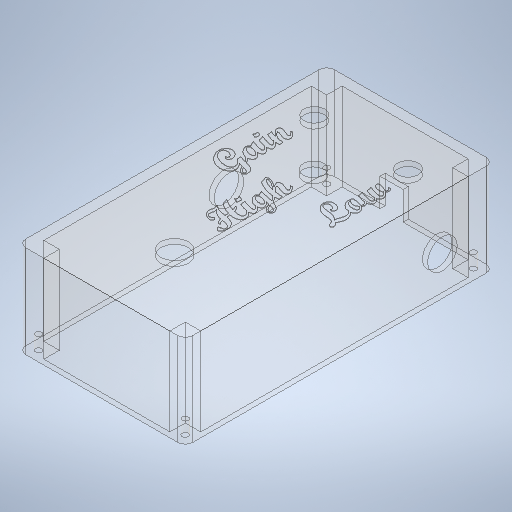
# Autodesk Inventor part: obudowa
Saved by Autodesk Inventor 2025 (Build 290162000, 162)
## iProperties
Created: 2026-04-02
Part Number: obudowa
Material: Tworzywo sztuczne PET
Document SubType Name: Modeling
Designer: zzapa
Density: 1.541 g/cm^3
Appearance: Poliwęglan — przezroczysty
Author: zzapa
Autodesk Inventor part; units mm, degrees
ref_plane "YZ Plane" through (0, 0, 0) normal (1, 0, 0) x (0, 1, 0)
ref_plane "XZ Plane" through (0, 0, 0) normal (0, 1, 0) x (-1, 0, 0)
ref_plane "XY Plane" through (0, 0, 0) normal (0, 0, 1) x (1, 0, 0)
sketch "Szkic1" plane through (0, 0, 0) normal (0, 1, 0) x (-1, 0, 0)
  line L0 (65, -120) -> (0, -120)
  line L1 (0, -120) -> (0, 0)
  line L2 (0, 0) -> (65, 0)
  line L3 (65, 0) -> (65, -120)
  dimension "d0" = 120
  dimension "d1" = 65
  constraints: 8 end point, 2 parallel, 1 coincident, 1 horizontal, 1 perpendicular
  measures "d0" distance of L2.end L0.start
  measures "d1" distance of L0.start L0.end
extrude "Gabaryt" add sketch "Szkic1" along normal blind 36
ref_plane "Konstrukcja wycięcia" through (0, 34, 0) normal (0, 1, 0) x (1, 0, 0)
sketch "Szkic2" plane through (0, 0, 0) normal (0, -1, 0) x (1, 0, 0)
  line L0 (-65, 0) -> (0, 0) projected
  line L1 (-65, -120) -> (-65, 0) projected
  line L2 (0, -120) -> (-65, -120) projected
  line L3 (0, 0) -> (0, -120) projected
  line L4 (-2, -118) -> (-63, -118)
  line L5 (-63, -118) -> (-63, -2)
  line L6 (-63, -2) -> (-2, -2)
  line L7 (-2, -2) -> (-2, -118)
  dimension "d4" = 2
  constraints: 8 end point, 3 other
  measures "d4" distance between parallel lines of L3 L7
extrude "Wydrążenie" cut sketch "Szkic2" against normal up to surface (34 mm away) contours L4 L5 L6 L7
sketch "Szkic6" plane through (0, 0, 0) normal (0, -1, 0) x (1, 0, 0)
  line L0 (-65, 0) -> (0, 0) projected
  line L1 (-8, -8) -> (0, -8)
  line L2 (0, -8) -> (0, 0)
  line L3 (0, 0) -> (-8, 0)
  line L4 (-8, 0) -> (-8, -8)
  line L5 (0, 0) -> (0, -120) projected
  line L6 (0, -120) -> (-65, -120) projected
  line L7 (-65, -120) -> (-65, 0) projected
  line L8 (0, 0) -> (0, -120) projected
  line L9 (0, -60) -> (-65, -60)
  line L10 (-32.5, 0) -> (-32.5, -120)
  line L11 (-57, -8) -> (-65, -8)
  line L12 (-65, -8) -> (-65, 0)
  line L13 (-65, 0) -> (-57, 0)
  line L14 (-57, 0) -> (-57, -8)
  line L15 (-8, -112) -> (0, -112)
  line L16 (0, -112) -> (0, -120)
  line L17 (0, -120) -> (-8, -120)
  line L18 (-8, -120) -> (-8, -112)
  line L19 (-57, -112) -> (-65, -112)
  line L20 (-65, -112) -> (-65, -120)
  line L21 (-65, -120) -> (-57, -120)
  line L22 (-57, -120) -> (-57, -112)
  point P0 (-57, -120)
  point P1 (-65, -112)
  point P2 (-57, 0)
  point P3 (-8, -120)
  point P4 (0, -112)
  point P5 (-8, 0)
  dimension "d16" = 8
  dimension "d17" = 8
  constraints: 36 end point, 9 symmetric about line, 4 midpoint, 2 parallel, 1 horizontal, 1 perpendicular
  measures "d16" distance of L1.start L1.end
  measures "d17" distance of L3.end L1.start
extrude "Materiał na insert" add sketch "Szkic6" against normal up to surface (34 mm away) contours L0 L14 L11 L7 | L0 L2 L1 L4 | L19 L22 L6 L7 | L5 L6 L18 L15
sketch "Szkic7" plane through (0, 0, 0) normal (0, -1, 0) x (1, 0, 0)
  line L0 (0, 0) -> (0, -120) projected
  line L1 (0, -60) -> (-65, -60)
  line L2 (-65, -120) -> (-65, 0) projected
  line L3 (0, -120) -> (-65, -120) projected
  line L4 (-32.5, -120) -> (-32.5, 0)
  line L5 (-65, 0) -> (0, 0) projected
  point P0 (-4, -4)
  point P1 (-61, -4)
  point P2 (-4, -116)
  point P3 (-61, -116)
  dimension "d20" = 4
  dimension "d21" = 4
  constraints: 4 end point, 4 midpoint, 3 symmetric about line
  measures "d20" horizontal distance of L0.start point (-4, -4)
  measures "d21" horizontal distance of point (-4, -4) L0.start
hole "Otwory montażowe" at (-4, 0, -4) at (-61, 0, -4) at (-4, 0, -116) at (-61, 0, -116) direction (0, 1, 0) diameter 2.4 depth 5.5
fillet "Zaokrąglenie1" radius 3 4 edges at (-65, 18, 0) (0, 18, 0) (0, 18, -120) (-65, 18, -120)
sketch "Szkic8" plane through (-65, 0, -117) normal (-1, 0, 0) x (0, 0, 1)
  line L0 (-3, 36) -> (-3, 0) projected
  line L1 (0, 0) -> (114, 0) projected
  line L2 (0, 0) -> (-3, 0) projected
  line L3 (117, 0) -> (117, 36) projected
  point P0 (37, 15)
  dimension "d30" = 15
  dimension "d39" = 80
  measures "d30" distance from line of L1 point (37, 15)
  measures "d39" distance from line of L3 point (37, 15)
hole "JACK 1" at (-65, 15, -80) direction (1, 0, 0) diameter 11.5 depth 2
sketch "Szkic9" plane through (0, 0, -3) normal (1, 0, 0) x (0, 0, -1)
  line L0 (0, 0) -> (114, 0) projected
  line L1 (-3, 36) -> (-3, 0) projected
  point P0 (97, 15)
  dimension "d40" = 15
  dimension "d41" = 100
  measures "d40" distance from line of L0 point (97, 15)
  measures "d41" distance from line of point (97, 15) L1
hole "JACK 2" at (0, 15, -100) direction (-1, 0, 0) diameter 11.5 end up to face face through (-2, 11.3333, -77.3333) facing (-1, 0, 0)
sketch "Szkic11" plane through (0, 36, 0) normal (0, 1, 0) x (1, 0, 0)
  circle A0 centre (-50.7217, 100.8782) radius 4
  circle A1 centre (-32.5, 82.3712) radius 4
  line L0 (-3, 120) -> (-62, 120) projected
  line L1 (-32.5, 120) -> (-32.5, 0)
  line L2 (-62, 0) -> (-3, 0) projected
  circle A2 centre (-14.2783, 100.8782) radius 4
  circle A3 centre (-32.5, 28.3603) radius 5.3281
  point P0 (0, 0)
  dimension "d51" = 8
  constraints: 4 centre point, 2 end point, 2 midpoint, 2 point on line, 1 equal radius, 1 symmetric about line, 1 other
  measures "d51" diameter of A0
extrude "Wyciągnięcie proste7" cut sketch "Szkic11" against normal up to surface (2 mm away)
sketch "Szkic12" plane through (-3, 0, -120) normal (0, 0, -1) x (-1, 0, 0)
  line L0 (0, 0) -> (59, 0) projected
  line L1 (30.3172, 11) -> (39.3172, 11)
  line L2 (39.3172, 11) -> (39.3172, 0)
  line L3 (39.3172, 0) -> (30.3172, 0)
  line L4 (30.3172, 0) -> (30.3172, 11)
  point P0 (-3, 0)
  point P1 (30.3172, 0)
  dimension "d54" = 11
  dimension "d55" = 9
  constraints: 8 end point, 2 parallel, 1 horizontal, 1 perpendicular, 1 point on line
  measures "d54" distance of L3.end L1.start
  measures "d55" distance of L1.start L1.end
extrude "Wyciągnięcie proste8" cut sketch "Szkic12" against normal up to surface (2 mm away)
sketch "Szkic13" plane through (0, 36, 0) normal (0, 1, 0) x (1, 0, 0)
  line L0 (-58.0791, 56.7666) -> (-58.0791, 90.8782) construction
  line L1 (-58.0791, 90.8782) -> (-43.3643, 90.8782) construction
  line L2 (-43.3643, 90.8782) -> (-43.3643, 56.7666) construction
  line L3 (-43.3643, 56.7666) -> (-58.0791, 56.7666) construction
  line L4 (-41.629, 38.2595) -> (-41.629, 72.3712) construction
  line L5 (-41.629, 72.3712) -> (-23.371, 72.3712) construction
  line L6 (-23.371, 72.3712) -> (-23.371, 38.2595) construction
  line L7 (-23.371, 38.2595) -> (-41.629, 38.2595) construction
  line L8 (-22.0376, 56.7666) -> (-22.0376, 90.8782) construction
  line L9 (-22.0376, 90.8782) -> (-6.519, 90.8782) construction
  line L10 (-6.519, 90.8782) -> (-6.519, 56.7666) construction
  line L11 (-6.519, 56.7666) -> (-22.0376, 56.7666) construction
  circle A0 centre (-50.7217, 100.8782) radius 4 projected
  circle A1 centre (-32.5, 82.3712) radius 4 projected
  circle A2 centre (-14.2783, 100.8782) radius 4 projected
  line L12 (-50.7217, 100.8782) -> (-50.7217, 90.8782)
  line L13 (-32.5, 82.3712) -> (-32.5, 72.3712)
  line L14 (-14.2783, 100.8782) -> (-14.2783, 90.8782)
  spline S0 degree 2 poles (-49.1006, 73.4653) (-48.5617, 73.001) (-47.8817, 71.6743) knots 0 0 0 1 1 1
  spline S1 degree 2 poles (-47.8817, 71.6743) (-46.0492, 71.4006) (-44.0426, 69.5101) (-44.0426, 68.3326) knots 0 0 0 1 2 2 2
  spline S2 degree 2 poles (-44.0426, 68.3326) (-44.0426, 67.7688) (-44.565, 67.1303) (-45.0293, 67.1303) knots 0 0 0 1 2 2 2
  spline S3 degree 2 poles (-45.0293, 67.1303) (-46.3146, 67.1303) (-47.5169, 69.6262) knots 0 0 0 1 1 1
  spline S4 degree 2 poles (-47.5169, 69.6262) (-48.4456, 69.8832) (-49.1836, 70.132) knots 0 0 0 1 1 1
  spline S5 degree 2 poles (-49.1836, 70.132) (-48.5617, 69.6925) (-47.5998, 68.0424) (-47.5998, 67.3293) knots 0 0 0 1 2 2 2
  spline S6 degree 2 poles (-47.5998, 67.3293) (-47.5998, 66.1685) (-49.6064, 64.6345) (-51.1404, 64.6345) knots 0 0 0 1 2 2 2
  spline S7 degree 2 poles (-51.1404, 64.6345) (-52.7574, 64.6345) (-55.6595, 66.3675) (-57.4008, 69.195) (-57.4008, 70.5134) knots 0 0 0 1 2 3 3 3
  spline S8 degree 2 poles (-57.4008, 70.5134) (-57.4008, 71.6991) (-56.0492, 73.1834) (-54.9713, 73.1834) knots 0 0 0 1 2 2 2
  spline S9 degree 2 poles (-54.9713, 73.1834) (-53.8187, 73.1834) (-52.0525, 71.5167) (-52.0525, 70.4388) knots 0 0 0 1 2 2 2
  spline S10 degree 2 poles (-52.0525, 70.4388) (-52.0525, 69.8003) (-52.6744, 68.9711) (-53.1222, 68.9711) knots 0 0 0 1 2 2 2
  spline S11 degree 2 poles (-53.1222, 68.9711) (-53.4041, 68.9711) (-53.827, 69.2945) (-53.827, 69.5101) knots 0 0 0 1 2 2 2
  spline S12 degree 2 poles (-53.827, 69.5101) (-53.827, 69.7174) (-53.5865, 69.7174) knots 0 0 0 1 1 1
  spline S13 degree 2 poles (-53.5865, 69.7174) (-53.371, 69.7174) (-53.1388, 70.0325) (-53.1388, 70.2398) knots 0 0 0 1 2 2 2
  spline S14 degree 2 poles (-53.1388, 70.2398) (-53.1388, 70.787) (-54.6479, 71.7986) (-55.5103, 71.7986) knots 0 0 0 1 2 2 2
  spline S15 degree 2 poles (-55.5103, 71.7986) (-56.1239, 71.7986) (-56.8867, 71.0109) (-56.8867, 70.3973) knots 0 0 0 1 2 2 2
  spline S16 degree 2 poles (-56.8867, 70.3973) (-56.8867, 69.4603) (-55.2366, 67.719) (-52.5418, 66.6245) (-51.3229, 66.6245) knots 0 0 0 1 2 3 3 3
  spline S17 degree 2 poles (-51.3229, 66.6245) (-50.2117, 66.6245) (-48.8933, 67.5864) (-48.8933, 68.3824) knots 0 0 0 1 2 2 2
  spline S18 degree 2 poles (-48.8933, 68.3824) (-48.8933, 69.734) (-50.8005, 70.9695) knots 0 0 0 1 1 1
  line L15 (-50.8005, 70.9695) -> (-50.9829, 72.263)
  spline S19 degree 2 poles (-50.9829, 72.263) (-51.0161, 72.5035) (-50.8668, 72.5035) knots 0 0 0 1 1 1
  spline S20 degree 2 poles (-50.8668, 72.5035) (-50.8005, 72.5035) (-49.7557, 72.1386) (-48.5285, 71.8152) knots 0 0 0 1 2 2 2
  spline S21 degree 2 poles (-48.5285, 71.8152) (-49.1421, 72.8849) (-49.8967, 73.4653) knots 0 0 0 1 1 1
  line L16 (-49.8967, 73.4653) -> (-49.1006, 73.4653)
  spline S22 degree 2 poles (-46.8204, 69.4603) (-45.9249, 67.6693) (-45.0542, 67.6693) knots 0 0 0 1 1 1
  spline S23 degree 2 poles (-45.0542, 67.6693) (-44.5899, 67.6693) (-44.5899, 68.1088) knots 0 0 0 1 1 1
  spline S24 degree 2 poles (-44.5899, 68.1088) (-44.5899, 68.9794) (-46.8204, 69.4603) knots 0 0 0 1 1 1
  spline S25 degree 2 poles (-49.1006, 80.8119) (-48.0559, 79.7091) (-47.4257, 78.7555) (-47.4257, 78.3243) knots 0 0 0 1 2 2 2
  spline S26 degree 2 poles (-47.4257, 78.3243) (-47.4257, 77.2381) (-49.3494, 77.2962) knots 0 0 0 1 1 1
  spline S27 degree 2 poles (-49.3494, 77.2962) (-48.3627, 76.6079) (-47.4257, 75.4471) (-47.4257, 74.8252) knots 0 0 0 1 2 2 2
  spline S28 degree 2 poles (-47.4257, 74.8252) (-47.4257, 74.2199) (-48.5617, 73.3741) (-49.3909, 73.3741) knots 0 0 0 1 2 2 2
  spline S29 degree 2 poles (-49.3909, 73.3741) (-50.419, 73.3741) (-52.293, 74.5101) (-53.4539, 76.2845) (-53.4539, 76.9645) knots 0 0 0 1 2 3 3 3
  spline S30 degree 2 poles (-53.4539, 76.9645) (-53.4539, 77.8268) (-52.6579, 78.1668) knots 0 0 0 1 1 1
  line L17 (-52.6579, 78.1668) -> (-53.4373, 79.5847)
  line L18 (-53.4373, 79.5847) -> (-53.4373, 79.9744)
  line L19 (-53.4373, 79.9744) -> (-51.4224, 79.3608)
  spline S31 degree 2 poles (-51.4224, 79.3608) (-49.8967, 78.8882) (-49.3328, 78.8882) knots 0 0 0 1 1 1
  spline S32 degree 2 poles (-49.3328, 78.8882) (-48.7441, 78.8882) (-48.7441, 79.3111) knots 0 0 0 1 1 1
  spline S33 degree 2 poles (-48.7441, 79.3111) (-48.7441, 79.5764) (-49.3162, 80.2232) (-49.8967, 80.8119) knots 0 0 0 1 2 2 2
  line L20 (-49.8967, 80.8119) -> (-49.1006, 80.8119)
  spline S34 degree 2 poles (-48.7275, 75.7704) (-48.7275, 76.4587) (-51.0741, 77.6776) (-52.0691, 77.6776) knots 0 0 0 1 2 2 2
  spline S35 degree 2 poles (-52.0691, 77.6776) (-52.4588, 77.6776) (-52.89, 77.3293) (-52.89, 77.0391) knots 0 0 0 1 2 2 2
  spline S36 degree 2 poles (-52.89, 77.0391) (-52.89, 76.3509) (-50.5434, 75.1237) (-49.565, 75.1237) knots 0 0 0 1 2 2 2
  spline S37 degree 2 poles (-49.565, 75.1237) (-49.1918, 75.1237) (-48.7275, 75.4885) (-48.7275, 75.7704) knots 0 0 0 1 2 2 2
  spline S38 degree 2 poles (-49.1006, 84.195) (-47.4091, 82.5864) (-47.4091, 81.7821) knots 0 0 0 1 1 1
  spline S39 degree 2 poles (-47.4091, 81.7821) (-47.4091, 81.3426) (-48.3129, 80.7373) (-48.9928, 80.7373) knots 0 0 0 1 2 2 2
  spline S40 degree 2 poles (-48.9928, 80.7373) (-50.4605, 80.7373) (-53.0559, 81.7323) knots 0 0 0 1 1 1
  line L21 (-53.0559, 81.7323) -> (-53.4207, 83.4819)
  line L22 (-53.4207, 83.4819) -> (-53.4207, 83.5648)
  line L23 (-53.4207, 83.5648) -> (-51.2648, 82.8766)
  spline S41 degree 2 poles (-51.2648, 82.8766) (-49.9298, 82.4454) (-49.3577, 82.4454) knots 0 0 0 1 1 1
  spline S42 degree 2 poles (-49.3577, 82.4454) (-49.1338, 82.4454) (-48.8519, 82.6444) (-48.8519, 82.7937) knots 0 0 0 1 2 2 2
  spline S43 degree 2 poles (-48.8519, 82.7937) (-48.8519, 83.0673) (-49.2416, 83.6063) (-49.8967, 84.195) knots 0 0 0 1 2 2 2
  line L24 (-49.8967, 84.195) -> (-49.1006, 84.195)
  spline S44 degree 2 poles (-56.1073, 84.054) (-54.4572, 84.054) (-54.4572, 82.8351) knots 0 0 0 1 1 1
  spline S45 degree 2 poles (-54.4572, 82.8351) (-54.4572, 82.2464) (-54.8137, 81.8235) knots 0 0 0 1 1 1
  spline S46 degree 2 poles (-54.8137, 81.8235) (-55.419, 82.2215) (-56.1736, 82.4454) knots 0 0 0 1 1 1
  spline S47 degree 2 poles (-56.1736, 82.4454) (-55.8419, 82.9844) (-55.8419, 83.3161) knots 0 0 0 1 1 1
  spline S48 degree 2 poles (-55.8419, 83.3161) (-55.8419, 83.6892) (-56.1073, 84.054) knots 0 0 0 1 1 1
  spline S49 degree 2 poles (-49.1089, 90.9612) (-47.4257, 89.3691) (-47.4257, 88.2331) knots 0 0 0 1 1 1
  spline S50 degree 2 poles (-47.4257, 88.2331) (-47.4257, 87.7688) (-48.0724, 87.2049) (-48.6197, 87.2049) knots 0 0 0 1 2 2 2
  spline S51 degree 2 poles (-48.6197, 87.2049) (-49.3577, 87.2049) (-50.8668, 87.8102) knots 0 0 0 1 1 1
  spline S52 degree 2 poles (-50.8668, 87.8102) (-51.6794, 88.1336) (-51.895, 88.1336) knots 0 0 0 1 1 1
  spline S53 degree 2 poles (-51.895, 88.1336) (-52.1189, 88.1336) (-52.1189, 87.9595) knots 0 0 0 1 1 1
  spline S54 degree 2 poles (-52.1189, 87.9595) (-52.1189, 87.8683) (-52.0194, 87.7107) knots 0 0 0 1 1 1
  spline S55 degree 2 poles (-52.0194, 87.7107) (-51.9282, 87.5615) (-51.754, 87.3708) knots 0 0 0 1 1 1
  spline S56 degree 2 poles (-51.754, 87.3708) (-51.5965, 87.1967) (-51.3643, 86.9894) knots 0 0 0 1 1 1
  spline S57 degree 2 poles (-51.3643, 86.9894) (-51.1736, 86.7986) (-50.9249, 86.5913) knots 0 0 0 1 1 1
  line L25 (-50.9249, 86.5913) -> (-50.4771, 86.2016)
  spline S58 degree 2 poles (-50.4771, 86.2016) (-50.1703, 85.9529) (-49.822, 85.8865) knots 0 0 0 1 1 1
  spline S59 degree 2 poles (-49.822, 85.8865) (-49.2416, 85.787) (-48.7524, 85.7456) knots 0 0 0 1 1 1
  spline S60 degree 2 poles (-48.7524, 85.7456) (-48.3875, 85.729) (-47.7656, 85.729) knots 0 0 0 1 1 1
  line L26 (-47.7656, 85.729) -> (-47.4091, 84.2033)
  spline S61 degree 2 poles (-47.4091, 84.2033) (-48.3378, 84.1287) (-48.7938, 84.1287) knots 0 0 0 1 1 1
  spline S62 degree 2 poles (-48.7938, 84.1287) (-49.9049, 84.1287) (-51.8867, 84.6428) (-53.1305, 85.2149) knots 0 0 0 1 2 2 2
  line L27 (-53.1305, 85.2149) -> (-53.4539, 86.8981)
  spline S63 degree 2 poles (-53.4539, 86.8981) (-52.0277, 86.3675) (-51.2068, 86.2016) knots 0 0 0 1 1 1
  spline S64 degree 2 poles (-51.2068, 86.2016) (-52.4671, 87.3293) (-53.4373, 88.656) (-53.4373, 89.1784) knots 0 0 0 1 2 2 2
  spline S65 degree 2 poles (-53.4373, 89.1784) (-53.4373, 89.5267) (-52.9066, 89.991) (-52.5086, 89.991) knots 0 0 0 1 2 2 2
  spline S66 degree 2 poles (-52.5086, 89.991) (-51.8452, 89.991) (-50.3361, 89.4023) knots 0 0 0 1 1 1
  spline S67 degree 2 poles (-50.3361, 89.4023) (-49.2914, 88.9877) (-48.9846, 88.9877) knots 0 0 0 1 1 1
  spline S68 degree 2 poles (-48.9846, 88.9877) (-48.57, 88.9877) (-48.57, 89.3277) knots 0 0 0 1 1 1
  spline S69 degree 2 poles (-48.57, 89.3277) (-48.57, 89.8335) (-49.8967, 90.9612) knots 0 0 0 1 1 1
  line L28 (-49.8967, 90.9612) -> (-49.1089, 90.9612)
  spline S70 degree 2 poles (-30.8541, 55.5553) (-29.9834, 54.7178) (-29.1708, 53.3413) (-29.1708, 52.6199) knots 0 0 0 1 2 2 2
  spline S71 degree 2 poles (-29.1708, 52.6199) (-29.1708, 51.8073) (-30.6053, 50.6962) (-31.9818, 50.6962) knots 0 0 0 1 2 2 2
  spline S72 degree 2 poles (-31.9818, 50.6962) (-32.5539, 50.6962) (-33.4826, 50.8455) knots 0 0 0 1 1 1
  spline S73 degree 2 poles (-33.4826, 50.8455) (-33.3997, 49.809) (-33.3831, 49.5768) knots 0 0 0 1 1 1
  spline S74 degree 2 poles (-33.3831, 49.5768) (-31.1111, 49.1374) (-29.1708, 46.9566) (-29.1708, 45.5719) knots 0 0 0 1 2 2 2
  spline S75 degree 2 poles (-29.1708, 45.5719) (-29.1708, 44.552) (-30.1161, 43.2335) (-30.5556, 43.2335) knots 0 0 0 1 2 2 2
  spline S76 degree 2 poles (-30.5556, 43.2335) (-30.8789, 43.2335) (-31.7081, 44.2203) (-31.7081, 44.411) knots 0 0 0 1 2 2 2
  spline S77 degree 2 poles (-31.7081, 44.411) (-31.7081, 44.6763) (-31.1277, 44.6763) knots 0 0 0 1 1 1
  spline S78 degree 2 poles (-31.1277, 44.6763) (-29.7098, 44.6763) (-29.7098, 45.6299) knots 0 0 0 1 1 1
  spline S79 degree 2 poles (-29.7098, 45.6299) (-29.7098, 46.3347) (-31.2769, 47.2634) (-33.1012, 47.5453) knots 0 0 0 1 2 2 2
  spline S80 degree 2 poles (-33.1012, 47.5453) (-32.9851, 46.7161) (-32.2968, 45.9035) knots 0 0 0 1 1 1
  spline S81 degree 2 poles (-32.2968, 45.9035) (-32.3715, 45.8455) (-32.8856, 45.804) knots 0 0 0 1 1 1
  spline S82 degree 2 poles (-32.8856, 45.804) (-33.6899, 46.5254) (-34.005, 47.7194) knots 0 0 0 1 1 1
  spline S83 degree 2 poles (-34.005, 47.7194) (-35.1161, 47.9599) (-36.5257, 48.6896) (-37.9934, 50.1821) knots 0 0 0 1 2 2 2
  spline S84 degree 2 poles (-37.9934, 50.1821) (-37.7114, 49.4607) (-37.7114, 49.0047) knots 0 0 0 1 1 1
  spline S85 degree 2 poles (-37.7114, 49.0047) (-37.7114, 48.7145) (-38.0265, 47.8272) (-38.0265, 47.5536) knots 0 0 0 1 2 2 2
  spline S86 degree 2 poles (-38.0265, 47.5536) (-38.0265, 46.9732) (-37.1808, 46.2269) (-36.7413, 46.2269) knots 0 0 0 1 2 2 2
  spline S87 degree 2 poles (-36.7413, 46.2269) (-36.3018, 46.2269) (-35.937, 46.6913) knots 0 0 0 1 1 1
  spline S88 degree 2 poles (-35.937, 46.6913) (-35.8043, 46.9068) (-35.6882, 46.9068) knots 0 0 0 1 1 1
  spline S89 degree 2 poles (-35.6882, 46.9068) (-35.4809, 46.9068) (-34.8673, 46.3513) (-34.8673, 46.1108) knots 0 0 0 1 2 2 2
  spline S90 degree 2 poles (-34.8673, 46.1108) (-34.8673, 45.8455) (-35.6302, 45.3894) (-36.0945, 45.3894) knots 0 0 0 1 2 2 2
  spline S91 degree 2 poles (-36.0945, 45.3894) (-37.1144, 45.3894) (-39.1625, 47.3878) (-39.1625, 48.3745) knots 0 0 0 1 2 2 2
  spline S92 degree 2 poles (-39.1625, 48.3745) (-39.1625, 48.5901) (-38.8143, 49.809) (-38.8143, 50.0329) knots 0 0 0 1 2 2 2
  spline S93 degree 2 poles (-38.8143, 50.0329) (-38.8143, 50.4723) (-39.1957, 50.8952) knots 0 0 0 1 1 1
  spline S94 degree 2 poles (-39.1957, 50.8952) (-38.9221, 51.4176) (-38.8474, 51.4176) knots 0 0 0 1 1 1
  spline S95 degree 2 poles (-38.8474, 51.4176) (-38.7562, 51.4176) (-37.9187, 50.5884) (-36.3765, 50.0578) (-34.2703, 49.7675) knots 0 0 0 1 2 3 3 3
  spline S96 degree 2 poles (-34.2703, 49.7675) (-34.3035, 50.5553) (-34.3947, 51.144) knots 0 0 0 1 1 1
  spline S97 degree 2 poles (-34.3947, 51.144) (-35.4643, 51.4508) (-36.9237, 52.1805) (-38.408, 53.1257) (-38.7313, 53.6316) (-39.1625, 55.2568) (-39.1625, 55.2651) knots 0 0 0 1 2 3 4 5 5 5
  spline S98 degree 2 poles (-39.1625, 55.2651) (-39.1625, 55.348) (-39.1211, 55.348) knots 0 0 0 1 1 1
  spline S99 degree 2 poles (-39.1211, 55.348) (-39.0216, 55.348) (-38.1592, 54.7261) (-35.9204, 53.5652) (-34.6517, 53.1755) knots 0 0 0 1 2 3 3 3
  spline S100 degree 2 poles (-34.6517, 53.1755) (-34.7678, 53.9218) (-35.3068, 54.6929) knots 0 0 0 1 1 1
  spline S101 degree 2 poles (-35.3068, 54.6929) (-35.2653, 54.7841) (-35.1078, 54.8256) (-34.7927, 54.8256) knots 0 0 0 1 2 2 2
  spline S102 degree 2 poles (-34.7927, 54.8256) (-34.0796, 54.2369) (-33.7811, 52.9267) knots 0 0 0 1 1 1
  spline S103 degree 2 poles (-33.7811, 52.9267) (-32.4295, 52.6365) (-31.874, 52.6365) knots 0 0 0 1 1 1
  spline S104 degree 2 poles (-31.874, 52.6365) (-31.194, 52.6365) (-30.4063, 53.2253) (-30.4063, 53.7228) knots 0 0 0 1 2 2 2
  spline S105 degree 2 poles (-30.4063, 53.7228) (-30.4063, 54.1208) (-30.9204, 54.9251) (-31.6501, 55.5553) knots 0 0 0 1 2 2 2
  line L29 (-31.6501, 55.5553) -> (-30.8541, 55.5553)
  spline S106 degree 2 poles (-30.8624, 58.9301) (-29.1708, 57.3214) (-29.1708, 56.5171) knots 0 0 0 1 1 1
  spline S107 degree 2 poles (-29.1708, 56.5171) (-29.1708, 56.0777) (-30.0746, 55.4723) (-30.7546, 55.4723) knots 0 0 0 1 2 2 2
  spline S108 degree 2 poles (-30.7546, 55.4723) (-32.2222, 55.4723) (-34.8176, 56.4674) knots 0 0 0 1 1 1
  line L30 (-34.8176, 56.4674) -> (-35.1824, 58.217)
  line L31 (-35.1824, 58.217) -> (-35.1824, 58.2999)
  line L32 (-35.1824, 58.2999) -> (-33.0265, 57.6117)
  spline S109 degree 2 poles (-33.0265, 57.6117) (-31.6915, 57.1805) (-31.1194, 57.1805) knots 0 0 0 1 1 1
  spline S110 degree 2 poles (-31.1194, 57.1805) (-30.8955, 57.1805) (-30.6136, 57.3795) (-30.6136, 57.5287) knots 0 0 0 1 2 2 2
  spline S111 degree 2 poles (-30.6136, 57.5287) (-30.6136, 57.8024) (-31.0033, 58.3413) (-31.6584, 58.9301) knots 0 0 0 1 2 2 2
  line L33 (-31.6584, 58.9301) -> (-30.8624, 58.9301)
  spline S112 degree 2 poles (-37.869, 58.7891) (-36.2189, 58.7891) (-36.2189, 57.5702) knots 0 0 0 1 1 1
  spline S113 degree 2 poles (-36.2189, 57.5702) (-36.2189, 56.9815) (-36.5755, 56.5586) knots 0 0 0 1 1 1
  spline S114 degree 2 poles (-36.5755, 56.5586) (-37.1808, 56.9566) (-37.9353, 57.1805) knots 0 0 0 1 1 1
  spline S115 degree 2 poles (-37.9353, 57.1805) (-37.6036, 57.7194) (-37.6036, 58.0511) knots 0 0 0 1 1 1
  spline S116 degree 2 poles (-37.6036, 58.0511) (-37.6036, 58.4243) (-37.869, 58.7891) knots 0 0 0 1 1 1
  spline S117 degree 2 poles (-30.8624, 65.6962) (-29.9502, 64.8173) (-29.5191, 63.5984) knots 0 0 0 1 1 1
  spline S118 degree 2 poles (-29.5191, 63.5984) (-27.7363, 63.0262) (-25.8043, 61.2684) (-25.8043, 60.2899) knots 0 0 0 1 2 2 2
  spline S119 degree 2 poles (-25.8043, 60.2899) (-25.8043, 59.751) (-26.476, 59.0876) (-27.0315, 59.0876) knots 0 0 0 1 2 2 2
  spline S120 degree 2 poles (-27.0315, 59.0876) (-27.7695, 59.0876) (-28.9386, 60.406) (-29.4859, 61.9815) knots 0 0 0 1 2 2 2
  line L34 (-29.4859, 61.9815) -> (-30.8458, 62.28)
  spline S121 degree 2 poles (-30.8458, 62.28) (-30.0995, 61.6166) (-29.403, 60.6548) (-29.403, 60.1655) knots 0 0 0 1 2 2 2
  spline S122 degree 2 poles (-29.403, 60.1655) (-29.403, 59.5934) (-30.4809, 58.8637) (-31.335, 58.8637) knots 0 0 0 1 2 2 2
  spline S123 degree 2 poles (-31.335, 58.8637) (-32.7446, 58.8637) (-35.199, 61.003) (-35.199, 62.2136) knots 0 0 0 1 2 2 2
  spline S124 degree 2 poles (-35.199, 62.2136) (-35.199, 62.877) (-34.6352, 63.3911) knots 0 0 0 1 1 1
  spline S125 degree 2 poles (-34.6352, 63.3911) (-34.743, 63.7062) (-34.9668, 64.2037) knots 0 0 0 1 1 1
  line L35 (-34.9668, 64.2037) -> (-35.1824, 64.6929)
  line L36 (-35.1824, 64.6929) -> (-35.1824, 64.8505)
  spline S126 degree 2 poles (-35.1824, 64.8505) (-34.3698, 64.5768) (-33.5987, 64.4359) knots 0 0 0 1 1 1
  line L37 (-33.5987, 64.4359) -> (-30.1493, 63.7891)
  spline S127 degree 2 poles (-30.1493, 63.7891) (-30.4975, 64.7178) (-31.6584, 65.6962) knots 0 0 0 1 1 1
  line L38 (-31.6584, 65.6962) -> (-30.8624, 65.6962)
  spline S128 degree 2 poles (-30.6468, 61.2601) (-30.6468, 61.7493) (-31.7993, 62.5039) (-33.5738, 62.9267) (-33.9221, 62.9267) knots 0 0 0 1 2 3 3 3
  spline S129 degree 2 poles (-33.9221, 62.9267) (-34.2371, 62.9267) (-34.66, 62.6034) (-34.66, 62.3629) knots 0 0 0 1 2 2 2
  spline S130 degree 2 poles (-34.66, 62.3629) (-34.66, 61.6332) (-32.6949, 60.547) (-31.675, 60.547) knots 0 0 0 1 2 2 2
  spline S131 degree 2 poles (-31.675, 60.547) (-31.2023, 60.547) (-30.6468, 60.9367) (-30.6468, 61.2601) knots 0 0 0 1 2 2 2
  spline S132 degree 2 poles (-28.8723, 61.8405) (-28.0763, 59.61) (-27.0315, 59.61) knots 0 0 0 1 1 1
  spline S133 degree 2 poles (-27.0315, 59.61) (-26.7164, 59.61) (-26.3267, 59.9831) (-26.3267, 60.2733) knots 0 0 0 1 2 2 2
  spline S134 degree 2 poles (-26.3267, 60.2733) (-26.3267, 60.7709) (-27.5788, 61.5005) (-28.8723, 61.8405) knots 0 0 0 1 2 2 2
  spline S135 degree 2 poles (-30.8624, 72.4541) (-29.1708, 70.8206) (-29.1708, 69.7675) knots 0 0 0 1 1 1
  spline S136 degree 2 poles (-29.1708, 69.7675) (-29.1708, 69.3032) (-29.8093, 68.6896) (-30.2985, 68.6896) knots 0 0 0 1 2 2 2
  spline S137 degree 2 poles (-30.2985, 68.6896) (-31.1277, 68.6896) (-32.6285, 69.3198) knots 0 0 0 1 1 1
  spline S138 degree 2 poles (-32.6285, 69.3198) (-33.4411, 69.6597) (-33.6899, 69.6597) knots 0 0 0 1 1 1
  spline S139 degree 2 poles (-33.6899, 69.6597) (-33.9718, 69.6597) (-33.9718, 69.3944) knots 0 0 0 1 1 1
  spline S140 degree 2 poles (-33.9718, 69.3944) (-33.9718, 69.1125) (-33.2255, 68.0677) (-32.5788, 67.4873) knots 0 0 0 1 2 2 2
  spline S141 degree 2 poles (-32.5788, 67.4873) (-31.3101, 67.2468) (-29.5274, 67.2468) knots 0 0 0 1 1 1
  line L39 (-29.5274, 67.2468) -> (-29.1708, 65.7128)
  spline S142 degree 2 poles (-29.1708, 65.7128) (-29.8922, 65.6216) (-30.738, 65.6216) knots 0 0 0 1 1 1
  spline S143 degree 2 poles (-30.738, 65.6216) (-32.7944, 65.6216) (-36.335, 66.7493) (-38.3167, 67.9599) knots 0 0 0 1 2 2 2
  spline S144 degree 2 poles (-38.3167, 67.9599) (-38.6816, 68.8637) (-39.1459, 70.207) (-39.1459, 70.2982) knots 0 0 0 1 2 2 2
  spline S145 degree 2 poles (-39.1459, 70.2982) (-39.1459, 70.4806) (-38.5655, 70.7294) (-38.1343, 70.7294) knots 0 0 0 1 2 2 2
  spline S146 degree 2 poles (-38.1343, 70.7294) (-37.4046, 70.7294) (-35.6302, 69.8339) (-34.3781, 68.8803) knots 0 0 0 1 2 2 2
  spline S147 degree 2 poles (-34.3781, 68.8803) (-34.9088, 69.8007) (-35.1824, 70.406) (-35.1824, 70.7294) knots 0 0 0 1 2 2 2
  spline S148 degree 2 poles (-35.1824, 70.7294) (-35.1824, 71.0777) (-34.6766, 71.5171) (-34.262, 71.5171) knots 0 0 0 1 2 2 2
  spline S149 degree 2 poles (-34.262, 71.5171) (-33.6401, 71.5171) (-31.0448, 70.5221) (-30.7131, 70.5221) knots 0 0 0 1 2 2 2
  spline S150 degree 2 poles (-30.7131, 70.5221) (-30.5638, 70.5221) (-30.3317, 70.7045) (-30.3317, 70.8289) knots 0 0 0 1 2 2 2
  spline S151 degree 2 poles (-30.3317, 70.8289) (-30.3317, 71.2684) (-31.6584, 72.4541) knots 0 0 0 1 1 1
  line L40 (-31.6584, 72.4541) -> (-30.8624, 72.4541)
  spline S152 degree 2 poles (-33.6899, 67.678) (-36.5506, 70.1407) (-37.9022, 70.1407) knots 0 0 0 1 1 1
  spline S153 degree 2 poles (-37.9022, 70.1407) (-38.3167, 70.1407) (-38.3167, 69.9168) knots 0 0 0 1 1 1
  spline S154 degree 2 poles (-38.3167, 69.9168) (-38.3167, 69.5354) (-35.6053, 68.1257) (-33.6899, 67.678) knots 0 0 0 1 2 2 2
  spline S155 degree 2 poles (-10.974, 75.2398) (-9.3156, 73.6063) (-9.3156, 71.8981) knots 0 0 0 1 1 1
  spline S156 degree 2 poles (-9.3156, 71.8981) (-9.3156, 71.4006) (-9.5727, 70.4885) (-10.1697, 69.1701) (-10.3106, 68.6726) knots 0 0 0 1 2 3 3 3
  spline S157 degree 2 poles (-10.3106, 68.6726) (-9.2907, 67.7439) (-9.2907, 66.9894) knots 0 0 0 1 1 1
  spline S158 degree 2 poles (-9.2907, 66.9894) (-9.2907, 66.7323) (-9.639, 66.384) (-9.8795, 66.384) knots 0 0 0 1 2 2 2
  spline S159 degree 2 poles (-9.8795, 66.384) (-10.4018, 66.384) (-11.1979, 67.4122) (-11.3471, 68.3492) knots 0 0 0 1 2 2 2
  spline S160 degree 2 poles (-11.3471, 68.3492) (-11.8861, 68.7389) (-12.9143, 68.9628) (-14.0917, 69.0209) knots 0 0 0 1 2 2 2
  spline S161 degree 2 poles (-14.0917, 69.0209) (-16.513, 69.137) (-19.2659, 71.5001) (-19.2659, 72.8849) knots 0 0 0 1 2 2 2
  spline S162 degree 2 poles (-19.2659, 72.8849) (-19.2659, 73.8384) (-18.0635, 75.0573) (-17.1266, 75.0573) knots 0 0 0 1 2 2 2
  spline S163 degree 2 poles (-17.1266, 75.0573) (-16.0403, 75.0573) (-14.4151, 73.7804) (-14.4151, 72.9429) knots 0 0 0 1 2 2 2
  spline S164 degree 2 poles (-14.4151, 72.9429) (-14.4151, 72.5117) (-14.8878, 72.0142) (-15.3023, 72.0142) knots 0 0 0 1 2 2 2
  spline S165 degree 2 poles (-15.3023, 72.0142) (-15.5179, 72.0142) (-15.7999, 72.0971) knots 0 0 0 1 1 1
  spline S166 degree 2 poles (-15.7999, 72.0971) (-15.5843, 72.2796) (-15.5843, 72.5698) knots 0 0 0 1 1 1
  spline S167 degree 2 poles (-15.5843, 72.5698) (-15.5843, 73.0341) (-16.7037, 73.7389) (-17.4748, 73.7389) knots 0 0 0 1 2 2 2
  spline S168 degree 2 poles (-17.4748, 73.7389) (-18.0718, 73.7389) (-18.7518, 73.2) (-18.7518, 72.7273) knots 0 0 0 1 2 2 2
  spline S169 degree 2 poles (-18.7518, 72.7273) (-18.7518, 72.1635) (-17.9392, 71.5333) (-16.8032, 71.2845) (-14.2824, 71.0109) (-12.3339, 70.3559) (-11.3969, 69.452) knots 0 0 0 1 2 3 4 5 5 5
  spline S170 degree 2 poles (-11.3969, 69.452) (-11.4383, 70.0408) (-11.2227, 70.9031) (-10.6091, 72.5035) (-10.6091, 73.0839) knots 0 0 0 1 2 3 3 3
  spline S171 degree 2 poles (-10.6091, 73.0839) (-10.6091, 74.2116) (-11.77, 75.2398) knots 0 0 0 1 1 1
  line L41 (-11.77, 75.2398) -> (-10.974, 75.2398)
  spline S172 degree 2 poles (-10.9657, 81.4172) (-10.6589, 81.069) (-10.4101, 80.4056) (-10.4101, 80.2149) knots 0 0 0 1 2 2 2
  spline S173 degree 2 poles (-10.4101, 80.2149) (-10.4101, 79.7174) (-10.7916, 79.2282) knots 0 0 0 1 1 1
  spline S174 degree 2 poles (-10.7916, 79.2282) (-9.2907, 78.2331) (-9.2907, 76.9562) knots 0 0 0 1 1 1
  spline S175 degree 2 poles (-9.2907, 76.9562) (-9.2907, 76.1602) (-10.4931, 75.1651) (-11.4798, 75.1651) knots 0 0 0 1 2 2 2
  spline S176 degree 2 poles (-11.4798, 75.1651) (-13.047, 75.1651) (-15.3023, 77.3957) (-15.3023, 78.9462) knots 0 0 0 1 2 2 2
  spline S177 degree 2 poles (-15.3023, 78.9462) (-15.3023, 79.5267) (-15.0453, 80.0739) (-14.7053, 80.1983) (-14.44, 80.1983) knots 0 0 0 1 2 3 3 3
  spline S178 degree 2 poles (-14.44, 80.1983) (-13.1548, 80.1983) (-11.2808, 79.4935) knots 0 0 0 1 1 1
  spline S179 degree 2 poles (-11.2808, 79.4935) (-10.9574, 79.8501) (-10.9574, 80.2315) knots 0 0 0 1 1 1
  spline S180 degree 2 poles (-10.9574, 80.2315) (-10.9574, 80.6958) (-11.7617, 81.4172) knots 0 0 0 1 1 1
  line L42 (-11.7617, 81.4172) -> (-10.9657, 81.4172)
  spline S181 degree 2 poles (-14.8214, 79.1452) (-14.8629, 79.0374) (-14.8629, 78.8467) knots 0 0 0 1 1 1
  spline S182 degree 2 poles (-14.8629, 78.8467) (-14.8629, 77.9512) (-12.9889, 76.9396) (-11.7368, 76.9396) knots 0 0 0 1 2 2 2
  spline S183 degree 2 poles (-11.7368, 76.9396) (-11.0403, 76.9396) (-10.2692, 77.3791) (-10.2692, 77.7771) knots 0 0 0 1 2 2 2
  spline S184 degree 2 poles (-10.2692, 77.7771) (-10.2692, 78.2663) (-11.173, 78.8384) knots 0 0 0 1 1 1
  spline S185 degree 2 poles (-11.173, 78.8384) (-11.9856, 78.1834) (-12.9226, 78.1834) knots 0 0 0 1 1 1
  spline S186 degree 2 poles (-12.9226, 78.1834) (-14.0254, 78.1834) (-14.8214, 79.1452) knots 0 0 0 1 1 1
  spline S187 degree 2 poles (-10.9657, 90.9612) (-10.6921, 90.6295) (-10.4599, 89.9661) (-10.4599, 89.792) knots 0 0 0 1 2 2 2
  spline S188 degree 2 poles (-10.4599, 89.792) (-10.4599, 89.2862) (-10.8496, 88.8053) knots 0 0 0 1 1 1
  spline S189 degree 2 poles (-10.8496, 88.8053) (-9.2907, 87.5532) (-9.2907, 86.2265) knots 0 0 0 1 1 1
  spline S190 degree 2 poles (-9.2907, 86.2265) (-9.2907, 85.2481) (-10.3687, 84.8252) knots 0 0 0 1 1 1
  spline S191 degree 2 poles (-10.3687, 84.8252) (-9.2907, 83.9048) (-9.2907, 82.8351) knots 0 0 0 1 1 1
  spline S192 degree 2 poles (-9.2907, 82.8351) (-9.2907, 82.1386) (-10.2028, 81.3426) (-11.0154, 81.3426) knots 0 0 0 1 2 2 2
  spline S193 degree 2 poles (-11.0154, 81.3426) (-11.8778, 81.3426) (-13.6688, 81.8318) (-14.9624, 82.3376) knots 0 0 0 1 2 2 2
  line L43 (-14.9624, 82.3376) -> (-15.3023, 84.1452)
  line L44 (-15.3023, 84.1452) -> (-13.7684, 83.6394)
  spline S194 degree 2 poles (-13.7684, 83.6394) (-11.77, 82.9927) (-11.0072, 82.9927) knots 0 0 0 1 1 1
  spline S195 degree 2 poles (-11.0072, 82.9927) (-10.6506, 82.9927) (-10.1946, 83.3409) (-10.1946, 83.598) knots 0 0 0 1 2 2 2
  spline S196 degree 2 poles (-10.1946, 83.598) (-10.1946, 84.1535) (-11.0569, 84.7008) knots 0 0 0 1 1 1
  spline S197 degree 2 poles (-11.0569, 84.7008) (-12.1349, 84.7008) (-13.2957, 85.0905) knots 0 0 0 1 1 1
  line L45 (-13.2957, 85.0905) -> (-14.9624, 85.6544)
  line L46 (-14.9624, 85.6544) -> (-15.3023, 87.5117)
  line L47 (-15.3023, 87.5117) -> (-12.9226, 86.7323)
  spline S198 degree 2 poles (-12.9226, 86.7323) (-11.77, 86.3592) (-11.0984, 86.3592) knots 0 0 0 1 1 1
  spline S199 degree 2 poles (-11.0984, 86.3592) (-10.6921, 86.3592) (-10.2111, 86.7157) (-10.2111, 87.0142) knots 0 0 0 1 2 2 2
  spline S200 degree 2 poles (-10.2111, 87.0142) (-10.2111, 87.3791) (-10.7501, 88.0258) (-11.2974, 88.4321) knots 0 0 0 1 2 2 2
  spline S201 degree 2 poles (-11.2974, 88.4321) (-11.9607, 88.0673) (-12.6821, 88.0673) knots 0 0 0 1 1 1
  spline S202 degree 2 poles (-12.6821, 88.0673) (-13.7103, 88.0673) (-15.3023, 89.1038) (-15.3023, 89.7505) knots 0 0 0 1 2 2 2
  spline S203 degree 2 poles (-15.3023, 89.7505) (-15.3023, 90.1983) (-14.6307, 90.1983) knots 0 0 0 1 1 1
  spline S204 degree 2 poles (-14.6307, 90.1983) (-13.1713, 90.1983) (-11.3388, 89.0706) knots 0 0 0 1 1 1
  spline S205 degree 2 poles (-11.3388, 89.0706) (-11.0072, 89.4189) (-11.0072, 89.8003) knots 0 0 0 1 1 1
  spline S206 degree 2 poles (-11.0072, 89.8003) (-11.0072, 90.2646) (-11.7617, 90.9612) knots 0 0 0 1 1 1
  line L48 (-11.7617, 90.9612) -> (-10.9657, 90.9612)
  point P0 (0, 0)
  dimension "d60" = 10
  constraints: 6 end point, 3 midpoint, 3 vertical, 2 parallel, 1 perpendicular, 6 other
  measures "d60" distance of L12.start L12.end
extrude "Napisy" cut sketch "Szkic13" against normal blind 0.2 contours L16 S21 S29 S30 L17 L18 L19 S31 S32 S33 L20 S40 S25 S26 S27 S28 S0 | S0 S28 S29 S21 L16 | S0 S1 S2 S3 S4 S5 S6 S7 S8 S9 S10 S11 S12 S13 S14 S15 S16 S17 S18 L15 S19 S20 S21 S29 S28 | S40 L20 S25 | S25 L20 S40 L21 L22 L23 S41 S42 S43 S62 S38 S39 | S62 L24 S38 | S38 L24 S62 L27 S63 S64 S65 S66 S67 S68 S69 L28 S49 S50 S51 S52 S53 S54 S55 S56 S57 L25 S58 S59 S60 L26 S61 | S44 S45 S46 S47 S48 | L29 S105 S108 L30 L31 L32 S109 S110 S111 S123 S122 S106 S107 S70 | S70 S108 S105 L29 | S70 S71 S72 S73 S74 S75 S76 S77 S78 S79 S80 S81 S82 S83 S84 S85 S86 S87 S88 S89 S90 S91 S92 S93 S94 S95 S96 S97 S98 S99 S100 S101 S102 S103 S104 S105 S108 | S122 S123 S111 L33 S106 | S106 L33 S111 S123 S124 S125 L35 L36 S126 L37 S127 S143 S117 S118 S119 S120 L34 S121 S122 | S143 S127 L38 S117 | S117 L38 S127 S143 S144 S145 S146 S147 S148 S149 S150 S151 L40 S135 S136 S137 S138 S139 S140 S141 L39 S142 | S112 S113 S114 S115 S116 | L41 S171 S176 S177 S178 S179 S180 S193 S192 S172 S173 S174 S175 S155 | S155 S175 S176 S171 L41 | S155 S156 S157 S158 S159 S160 S161 S162 S163 S164 S165 S166 S167 S168 S169 S170 S171 S176 S175 | S192 S193 S180 L42 S172 | S172 L42 S180 S193 L43 L44 S194 S195 S196 S197 L45 L46 L47 S198 S199 S200 S201 S202 S203 S204 S205 S206 L48 S187 S188 S189 S190 S191 S192
equation "\"d0\" = obudowa_a"
equation "\"d1\" = obudowa_b"
equation "\"d2\" = obudowa_wys"
equation "\"d4\" = obudowa_grubosc"
equation "\"d6\" = obudowa_wys"
equation "\"d16\" = obudowa_otwory_montazowe_material_x"
equation "\"d17\" = obudowa_otwory_montazowe_material_y"
equation "\"d20\" = obudowa_otwory_montazowe_poz_x"
equation "\"d21\" = obudowa_otwory_montazowe_poz_y"
equation "\"d22\" = insert_D"
equation "\"d24\" = gniazdo_M2_D1"
equation "\"d25\" = gniazdo_M2_glebokosc"
equation "\"d27\" = insert_glebokosc"
equation "\"d29\" = obudowa_zaokraglenie"
equation "\"d30\" = obudowa_otwory_io1_wys"
equation "\"d39\" = obudowa_otwory_io1_poz"
equation "\"d32\" = obudowa_otwory_io1_D"
equation "\"d37\" = insert_glebokosc"
equation "\"d40\" = obudowa_otwory_io2_wys"
equation "\"d41\" = obudowa_otwory_io2_poz"
equation "\"d42\" = obudowa_otwory_io2_D"
equation "\"d51\" = obudowa_otwory_pot_D"
equation "\"d54\" = input_wys"
equation "\"d55\" = input_a"
equation "\"gniazdo_M2_glebokosc\" = 1.5"
equation "\"gniazdo_M2_D1\" = 4.5"
equation "\"gniazdo_M2_D2\" = 2.6"
equation "\"podstawa_b\" = 65"
equation "\"podstawa_wys\" = 2"
equation "\"podstawa_otwory_montazowe_poz_x\" = 4"
equation "\"podstawa_otwory_montazowe_poz_y\" = 4"
equation "\"obudowa_b\" = 65"
equation "\"obudowa_a\" = 120"
equation "\"obudowa_wys\" = 36"
equation "\"obudowa_grubosc\" = 2"
equation "\"d5\" = -obudowa_grubosc"
equation "\"obudowa_prowadnica_odsuniecie\" = 2"
equation "\"obudowa_prowadnica_grubosc\" = 2"
equation "\"obudowa_kontrolki_a\" = 38"
equation "\"obudowa_prowadnica_wys\" = 19"
equation "\"obudowa_otwory_montazowe_poz_y\" = 4"
equation "\"obudowa_otwory_montazowe_poz_x\" = 4"
equation "\"obudowa_otwory_montazowe_material_y\" = 8"
equation "\"obudowa_otwory_montazowe_material_x\" = 8"
equation "\"insert_D\" = 2.4"
equation "\"insert_glebokosc\" = 5.5"
equation "\"obudowa_zaokraglenie\" = 3"
equation "\"podstawa_zaokraglenie\" = 3"
equation "\"obudowa_otwory_io_wys\" = 15"
equation "\"obudowa_otwory_io_D\" = 15"
equation "\"obudowa_otwory_io1_poz\" = 80"
equation "\"obudowa_otwory_io1_wys\" = 15"
equation "\"obudowa_otwory_io1_D\" = 11.5"
equation "\"obudowa_otwory_io2_poz\" = 100"
equation "\"obudowa_otwory_io2_wys\" = 15"
equation "\"obudowa_otwory_io2_D\" = 11.5"
equation "\"obudowa_otwory_pot_D\" = 8"
equation "\"input_b\" = 14.4"
equation "\"input_wys\" = 11"
equation "\"input_a\" = 9"
